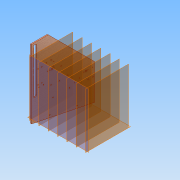
# Autodesk Inventor part: Selection_LHS
Saved by Autodesk Inventor 2018.1 (Build 221171000, 171)
## iProperties
Created: 2019-02-07
Part Number: Selection_LHS
Material: Wood (Oak)
Document SubType Name: Modeling
Designer: James
Density: 0.76 g/cm^3
Appearance: White Oak - Natural Medium Gloss
Author: James
Autodesk Inventor part; units mm, degrees
ref_plane "YZ Plane" through (0, 0, 0) normal (1, 0, 0) x (0, 1, 0)
ref_plane "XZ Plane" through (0, 0, 0) normal (0, 1, 0) x (-1, 0, 0)
ref_plane "XY Plane" through (0, 0, 0) normal (0, 0, 1) x (1, 0, 0)
derived "Selection_Skeleton.ipt"
ref_plane "Ground" through (0, 0, 0) normal (0, 1, 0) x (-1, 0, 0)
ref_plane "LHS inner" through (0, 0, 0) normal (1, 0, 0) x (0, 1, 0)
ref_plane "RHS inner" through (300, 0, 0) normal (1, 0, 0) x (0, 1, 0)
ref_plane "Lane 1" through (50, 0, 0) normal (1, 0, 0) x (0, 1, 0)
ref_plane "Lane 2" through (100, 0, 0) normal (1, 0, 0) x (0, 1, 0)
ref_plane "Lane 3" through (150, 0, 0) normal (1, 0, 0) x (0, 1, 0)
ref_plane "Lane 4" through (200, 0, 0) normal (1, 0, 0) x (0, 1, 0)
ref_plane "Lane 5" through (250, 0, 0) normal (1, 0, 0) x (0, 1, 0)
ref_plane "Back" through (0, 0, 0) normal (0, 0, 1) x (1, 0, 0)
sketch "Sketch1" plane through (0, 0, 0) normal (1, 0, 0) x (0, 1, 0)
  line L0 (-68, 0) -> (408, 0) projected
  line L1 (0, 408) -> (0, -68) projected
  line L2 (0, 0) -> (340, 0)
  line L3 (340, 0) -> (340, 340)
  line L4 (340, 340) -> (0, 340)
  line L5 (0, 340) -> (0, 0)
  dimension "d1" = 340
  dimension "d2" = 340
  constraints: 8 end point, 2 parallel, 1 horizontal, 1 perpendicular
  measures "d1" distance of L2.start L2.end
  measures "d2" distance of L2.end L3.end
extrude "Extrusion1" add sketch "Sketch1" against normal blind 5
chamfer "Chamfer1" distance 250 angle 45 1 edges at (-2.5, 340, 340)
sketch "Sketch2" plane through (-5, 0, 0) normal (-1, 0, 0) x (0, 0, 1)
  line L0 (0, 340) -> (0, 0) projected
  line L1 (0, 0) -> (340, 0) projected
  point P0 (35, 205)
  point P1 (99.2262, 195)
  point P2 (159.2262, 160)
  point P3 (95, 150)
  point P4 (35, 115)
  point P5 (99.2262, 105)
  dimension "d8" = 35
  dimension "d11" = 60
  dimension "d12" = 10
  dimension "d13" = 10
  dimension "d14" = 10
  dimension "d15" = 35
  dimension "d16" = 35
  dimension "d17" = 105
  dimension "d25" = 65
  dimension "d26" = 65
  dimension "d104" = 205
  constraints: 2 vertical alignment
  measures "d8" distance from line of point (35, 205) L0
  measures "d11" horizontal distance of point (159.226, 160) point (99.226, 195)
  measures "d12" vertical distance of point (99.226, 195) point (35, 205)
  measures "d13" vertical distance of point (159.226, 160) point (95, 150)
  measures "d14" vertical distance of point (99.226, 105) point (35, 115)
  measures "d15" vertical distance of point (159.226, 160) point (99.226, 195)
  measures "d16" vertical distance of point (95, 150) point (35, 115)
  measures "d17" distance from line of point (99.226, 105) L1
  measures "d25" distance of point (99.226, 195) point (35, 205)
  measures "d26" distance of point (159.226, 160) point (95, 150)
  measures "d104" distance from line of L1 point (35, 205)
hole "Ramp Holes" at (-5, 205, 35) at (-5, 195, 99.2262) at (-5, 160, 159.2262) at (-5, 150, 95) at (-5, 115, 35) at (-5, 105, 99.2262) direction (1, 0, 0) diameter 4.5 end through all clearance for "Socket Head Cap Screw" size "M4" standard "Ansi Metric M Profile"
sketch "Sketch3" plane through (-5, 0, 0) normal (-1, 0, 0) x (0, 0, 1)
  circle A0 centre (99.2262, 105) radius 2.25 projected
  circle A1 centre (35, 115) radius 2.25 projected
  point P0 (0, 0)
  point P1 (120, 65)
  point P2 (120, 40)
  dimension "d73" = 85
  dimension "d105" = 50
  dimension "d108" = 25
  constraints: 1 vertical alignment
  measures "d73" horizontal distance of A1.centre point (120, 65)
  measures "d105" vertical distance of point (120, 65) A1.centre
  measures "d108" distance of point (120, 40) point (120, 65)
hole "Hole2" at (-5, 65, 120) at (-5, 40, 120) direction (1, 0, 0) diameter 4.5 end through all clearance for "Socket Head Cap Screw" size "M4" standard "Ansi Metric M Profile"
sketch "Sketch4" plane through (-5, 0, 0) normal (-1, 0, 0) x (0, 0, 1)
  line L0 (0, 0) -> (340, 0) projected
  line L1 (0, 340) -> (0, 0) projected
  circle A0 centre (99.2262, 105) radius 2.25 projected
  circle A1 centre (35, 115) radius 2.25 projected
  point P0 (170, 110)
  dimension "d72" = 135
  dimension "d106" = 5
  measures "d72" horizontal distance of point (170, 110) A1.centre
  measures "d106" vertical distance of point (170, 110) A1.centre
hole "Hole3" at (-5, 110, 170) direction (1, 0, 0) diameter 8 end through all
sketch "Sketch5" plane through (-5, 0, 0) normal (-1, 0, 0) x (0, 0, 1)
  circle A0 centre (170, 110) radius 4 projected
  point P0 (0, 0)
  point P1 (170, 121)
  point P2 (170, 99)
  dimension "d46" = 22
  dimension "d47" = 11
  constraints: 2 vertical alignment
  measures "d46" distance of point (170, 99) point (170, 121)
  measures "d47" distance of A0.centre point (170, 121)
hole "Hole4" at (-5, 121, 170) at (-5, 99, 170) direction (1, 0, 0) diameter 3.4 end through all clearance for "Socket Head Cap Screw" size "M3" standard "Ansi Metric M Profile"
sketch "Sketch6" plane through (-5, 0, 0) normal (-1, 0, 0) x (0, 0, 1)
  circle A0 centre (170, 110) radius 4 projected
  point P0 (0, 0)
  point P1 (215, 105)
  point P2 (215, 80)
  dimension "d56" = 45
  dimension "d57" = 5
  dimension "d107" = 25
  constraints: 1 vertical alignment
  measures "d56" horizontal distance of point (215, 105) A0.centre
  measures "d57" vertical distance of point (215, 105) A0.centre
  measures "d107" distance of point (215, 105) point (215, 80)
hole "Hole5" at (-5, 105, 215) at (-5, 80, 215) direction (1, 0, 0) diameter 4.5 end through all clearance for "Socket Head Cap Screw" size "M4" standard "Ansi Metric M Profile"
sketch "Sketch8" plane through (-5, 0, 0) normal (-1, 0, 0) x (0, 0, 1)
  circle A0 centre (35, 205) radius 2.25 projected
  point P0 (0, 0)
  point P1 (25, 330)
  point P2 (25, 305)
  dimension "d74" = 25
  dimension "d75" = 100
  dimension "d84" = 10
  constraints: 1 vertical alignment
  measures "d74" distance of point (25, 305) point (25, 330)
  measures "d75" vertical distance of point (25, 305) A0.centre
  measures "d84" horizontal distance of A0.centre point (25, 305)
hole "Hole6" at (-5, 330, 25) at (-5, 305, 25) direction (1, 0, 0) diameter 4.5 end through all clearance for "Socket Head Cap Screw" size "M4" standard "Ansi Metric M Profile"
sketch "Sketch9" plane through (-5, 0, 0) normal (-1, 0, 0) x (0, 0, 1)
  circle A0 centre (25, 330) radius 2.25 projected
  line L0 (90, 340) -> (0, 340) projected
  point P0 (0, 0)
  point P1 (70, 327.5)
  dimension "d85" = 45
  dimension "d87" = 2.5
  measures "d85" horizontal distance of point (70, 327.5) A0.centre
  measures "d87" vertical distance of point (70, 327.5) A0.centre
hole "Hole7" at (-5, 327.5, 70) direction (1, 0, 0) diameter 3 end through all
sketch "Sketch10" plane through (-5, 0, 0) normal (-1, 0, 0) x (0, 0, 1)
  circle A0 centre (70, 327.5) radius 1.5 projected
  point P0 (0, 0)
  point P1 (70, 303.5)
  point P2 (70, 281.5)
  dimension "d95" = 24
  dimension "d96" = 22
  constraints: 2 vertical alignment
  measures "d95" distance of point (70, 303.5) A0.centre
  measures "d96" distance of point (70, 281.5) point (70, 303.5)
hole "Hole8" at (-5, 303.5, 70) at (-5, 281.5, 70) direction (1, 0, 0) diameter 3.4 end through all clearance for "Socket Head Cap Screw" size "M3" standard "Ansi Metric M Profile"
sketch "Sketch11" plane through (-5, 0, 0) normal (-1, 0, 0) x (0, 0, 1)
  circle A0 centre (170, 110) radius 4 projected
  point P0 (0, 0)
  point P1 (200, 120)
  dimension "d109" = 10
  dimension "d110" = 30
  measures "d109" vertical distance of point (200, 120) A0.centre
  measures "d110" horizontal distance of A0.centre point (200, 120)
hole "Hole9" at (-5, 120, 200) direction (1, 0, 0) diameter 3.4 end through all clearance for "Socket Head Cap Screw" size "M3" standard "Ansi Metric M Profile"
sketch "Sketch12" plane through (-5, 0, 0) normal (-1, 0, 0) x (0, 0, 1)
  circle A0 centre (170, 110) radius 4 projected
  point P0 (0, 0)
  point P1 (180, 117)
  point P2 (171, 88)
  dimension "d118" = 10
  dimension "d119" = 7
  dimension "d120" = 22
  dimension "d121" = 1
  measures "d118" horizontal distance of point (180, 117) A0.centre
  measures "d119" vertical distance of A0.centre point (180, 117)
  measures "d120" vertical distance of A0.centre point (171, 88)
  measures "d121" horizontal distance of A0.centre point (171, 88)
hole "Hole10" at (-5, 117, 180) at (-5, 88, 171) direction (1, 0, 0) diameter 4.5 end through all clearance for "Socket Head Cap Screw" size "M4" standard "Ansi Metric M Profile"
sketch "Sketch13" plane through (-5, 0, 0) normal (-1, 0, 0) x (0, 0, 1)
  circle A0 centre (70, 303.5) radius 1.7 projected
  circle A1 centre (70, 281.5) radius 1.7 projected
  point P0 (0, 0)
  point P1 (70, 292.5)
  dimension "d129" = 11
  dimension "d130" = 22
  constraints: 1 vertical alignment
  measures "d129" distance of point (70, 292.5) A0.centre
  measures "d130" distance of A0.centre A1.centre
hole "Hole11" at (-5, 292.5, 70) direction (1, 0, 0) diameter 8 end through all
sketch "Sketch14" plane through (-5, 0, 0) normal (-1, 0, 0) x (0, 0, 1)
  circle A0 centre (70, 292.5) radius 4 projected
  point P0 (0, 0)
  point P1 (55, 257.5)
  dimension "d138" = 35
  dimension "d139" = 15
  measures "d138" vertical distance of point (55, 257.5) A0.centre
  measures "d139" horizontal distance of point (55, 257.5) A0.centre
hole "Hole12" at (-5, 257.5, 55) direction (1, 0, 0) diameter 3.4 end through all clearance for "Socket Head Cap Screw" size "M3" standard "Ansi Metric M Profile"
sketch "Sketch15" plane through (-5, 0, 0) normal (-1, 0, 0) x (0, 0, 1)
  circle A0 centre (55, 257.5) radius 1.7 projected
  point P0 (0, 0)
  point P1 (45, 232.5)
  dimension "d147" = 25
  dimension "d148" = 10
  measures "d147" vertical distance of point (45, 232.5) A0.centre
  measures "d148" horizontal distance of point (45, 232.5) A0.centre
hole "Hole13" at (-5, 232.5, 45) direction (1, 0, 0) diameter 3.4 end through all clearance for "Socket Head Cap Screw" size "M3" standard "Ansi Metric M Profile"
sketch "Sketch17" plane through (-5, 0, 0) normal (-1, 0, 0) x (0, 0, 1)
  line L0 (92, 20) -> (323, 20) construction
  line L1 (92, 12.5) -> (323, 12.5)
  line L2 (323, 27.5) -> (92, 27.5)
  arc A0 (92, 27.5) -> (92, 12.5) centre (92, 20) ccw
  arc A1 (323, 12.5) -> (323, 27.5) centre (323, 20) ccw
  circle A2 centre (120, 40) radius 2.25 projected
  circle A3 centre (92, 18) radius 7.5
  circle A4 centre (192, 18) radius 7.5
  circle A5 centre (223, 18) radius 7.5
  circle A6 centre (323, 18) radius 7.5
  point P0 (0, 0)
  point P1 (207.5, 20)
  dimension "d156" = 231
  dimension "d157" = 15
  dimension "d158" = 20
  dimension "d163" = 28
  dimension "d164" = 15
  dimension "d165" = 15
  dimension "d166" = 15
  dimension "d167" = 15
  dimension "d168" = 2
  dimension "d169" = 100
  dimension "d170" = 100
  dimension "d171" = 131
  constraints: 8 end point, 6 centre point, 4 point on circle, 4 tangent, 3 horizontal alignment, 1 horizontal, 1 midpoint, 1 parallel, 1 vertical alignment
  measures "d156" distance of L0.start L0.end
  measures "d157" distance between parallel lines of L1 L2
  measures "d158" distance from line of A2.centre L0
  measures "d163" horizontal distance of L0.start A2.centre
  measures "d164" diameter of A3
  measures "d165" diameter of A4
  measures "d166" diameter of A5
  measures "d167" diameter of A6
  measures "d168" distance of L0.start A3.centre
  measures "d169" distance of A4.centre A3.centre
  measures "d170" distance of A6.centre A5.centre
  measures "d171" distance of A3.centre A5.centre
extrude "Extrusion3" cut sketch "Sketch17" against normal through all contours A0 A3 L1 | L1 A3 A0 | A3 A0 L2 A1 A6 L1 A5 A4 | A4 L1 | L1 A4 | A5 L1 | L1 A5 | A6 L1 A1 | A1 L1 A6
sketch "Sketch19" plane through (-5, 0, 0) normal (-1, 0, 0) x (0, 0, 1)
  line L0 (0, 0) -> (-30.8262, 0)
  line L1 (-30.8262, 0) -> (-100, 340)
  line L2 (0, 340) -> (90, 340) projected
  line L3 (-100, 340) -> (0, 340)
  line L4 (0, 0) -> (0, 340) projected
  line L5 (0, 340) -> (0, 0)
  dimension "d172" = 78.5
  dimension "d173" = 100
  constraints: 8 end point, 1 horizontal, 1 parallel, 1 perpendicular
  measures "d172" angle of L0 L1
  measures "d173" distance of L1.end L2.start
extrude "Extrusion4" add sketch "Sketch19" against normal up to surface (5 mm away)
sketch "Sketch20" plane through (-5, 0, 0) normal (-1, 0, 0) x (0, 0, 1)
  line L0 (-100, 340) -> (-30.8262, 0) projected
  line L1 (90, 340) -> (-100, 340) projected
  line L2 (-30.8262, 0) -> (340, 0) projected
  point P0 (0, 0)
  point P1 (-67.9159, 245)
  point P2 (-38.0108, 98.0113)
  dimension "d176" = 12.5
  dimension "d177" = 12.5
  dimension "d178" = 150
  dimension "d179" = 95
  dimension "d180" = 98.0113
  measures "d176" distance from line of L0 point (-67.916, 245)
  measures "d177" distance from line of point (-38.011, 98.011) L0
  measures "d178" distance of point (-38.011, 98.011) point (-67.916, 245)
  measures "d179" distance from line of L1 point (-67.916, 245)
  measures "d180" distance from line of L2 point (-38.011, 98.011)
hole "Hole14" at (-5, 245, -67.9159) at (-5, 98.0113, -38.0108) direction (1, 0, 0) diameter 4.5 end through all clearance for "Flat Head Machine Screw" size "M4" standard "Ansi Metric M Profile"
sketch "Sketch21" plane through (-5, 0, 0) normal (-1, 0, 0) x (0, 0, 1)
  line L0 (-30.8262, 0) -> (340, 0) projected
  circle A0 centre (120, 40) radius 2.25 projected
  point P0 (0, 0)
  point P1 (208, 35)
  point P2 (134, 35)
  point P3 (134, 55)
  point P4 (208, 55)
  dimension "d188" = 35
  dimension "d190" = 74
  dimension "d198" = 14
  dimension "d199" = 20
  constraints: 2 horizontal alignment, 2 vertical alignment
  measures "d188" distance from line of point (208, 35) L0
  measures "d190" distance of point (134, 35) point (208, 35)
  measures "d198" horizontal distance of A0.centre point (134, 35)
  measures "d199" distance of point (208, 35) point (208, 55)
hole "Hole15" at (-5, 35, 208) at (-5, 35, 134) at (-5, 55, 208) at (-5, 55, 134) direction (1, 0, 0) diameter 4.5 end through all clearance for "Flat Head Machine Screw" size "M4" standard "Ansi Metric M Profile"
equation "\"d13\" = d12"
equation "\"d14\" = d13"
equation "\"d16\" = d15"
equation "\"d26\" = d25"
equation "\"d47\" = 0.5 * d46"
equation "\"d129\" = 0.5 * d130"
equation "\"d164\" = d157"
equation "\"d165\" = d164"
equation "\"d166\" = d157"
equation "\"d167\" = d166"
equation "\"d170\" = d169"
equation "\"d177\" = d176"
body "Solid1"
